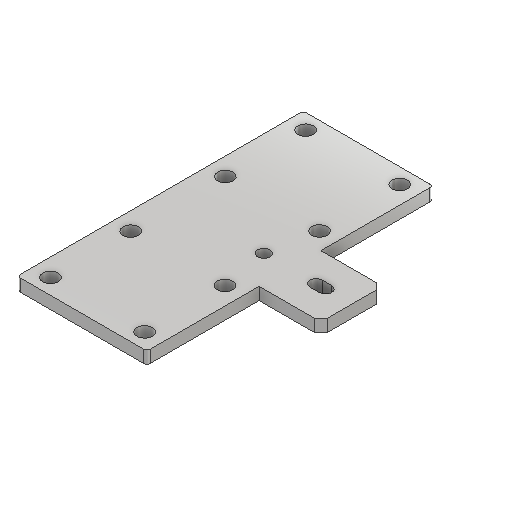
# Autodesk Inventor part: LC_ALU_4mm_X_End_Bearing_Side
Saved by Autodesk Inventor 2026.1 (Build 301233000, 233)
## iProperties
Created: 2017-05-25
Part Number: LC_ALU_4mm_X_End_Bearing_Side
Material: Ogólny
Document SubType Name: Modeling
Designer: Andrzej
Density: 1 g/cm^3
Appearance: Aluminium - ciemne
Mass: 16.3605 g
Surface Area: 100.28 cm^2
Volume: 16.3605 cm^3
Author: Andrzej
Autodesk Inventor part; units mm, degrees
ref_plane "YZ Plane" through (0, 0, 0) normal (1, 0, 0) x (0, 1, 0)
ref_plane "XZ Plane" through (0, 0, 0) normal (0, 1, 0) x (-1, 0, 0)
ref_plane "XY Plane" through (0, 0, 0) normal (0, 0, 1) x (1, 0, 0)
sketch "Szkic1" plane through (0, 0, 0) normal (0, 0, 1) x (1, 0, 0)
  line L0 (-10.2233, 17.3341) -> (-10.2233, -75.2659)
  line L1 (-10.2233, -75.2659) -> (31.7767, -75.2659)
  line L2 (-10.2233, 17.3341) -> (31.7767, 17.3341)
  line L3 (31.7767, 17.3341) -> (31.7767, -18.9659)
  line L4 (31.7767, -75.2659) -> (31.7767, -38.9659)
  line L5 (31.7767, -38.9659) -> (51.7767, -38.9659)
  line L6 (51.7767, -38.9659) -> (51.7767, -18.9659)
  line L7 (51.7767, -18.9659) -> (31.7767, -18.9659)
  line L8 (43.2767, -28.9659) -> (40.2767, -28.9659) construction
  line L9 (43.2767, -26.9659) -> (40.2767, -26.9659)
  line L10 (40.2767, -30.9659) -> (43.2767, -30.9659)
  arc A0 (43.2767, -30.9659) -> (43.2767, -26.9659) centre (43.2767, -28.9659) ccw
  arc A1 (40.2767, -26.9659) -> (40.2767, -30.9659) centre (40.2767, -28.9659) ccw
  point P0 (0, 0)
  point P1 (-4.4733, 12.3341)
  point P2 (26.0267, 12.3341)
  point P3 (-4.4733, -13.6659)
  point P4 (26.0267, -13.6659)
  point P5 (-4.4733, -44.2659)
  point P6 (26.0267, -44.2659)
  point P7 (-4.4733, -70.2659)
  point P8 (26.0267, -70.2659)
  point P9 (41.7767, -28.9659)
  point P10 (23.2767, -28.9659)
  dimension "d0" = 92.6
  dimension "d1" = 42
  dimension "d2" = 20
  dimension "d3" = 20
  dimension "d4" = 36.3
  dimension "d39" = 5
  dimension "d40" = 5
  dimension "d41" = 5
  dimension "d42" = 5
  dimension "d43" = 5.75
  dimension "d44" = 5.75
  dimension "d45" = 42
  dimension "d46" = 5.75
  dimension "d47" = 5.75
  dimension "d48" = 5.75
  dimension "d49" = 5.75
  dimension "d50" = 36.3
  dimension "d51" = 5.75
  dimension "d52" = 5.75
  dimension "d60" = 26
  dimension "d61" = 26
  dimension "d62" = 26
  dimension "d63" = 26
  dimension "d65" = 10
  dimension "d66" = 10
  dimension "d74" = 1.5
  dimension "d75" = 4
  dimension "d76" = 33.5
  dimension "d77" = 10
  constraints: 24 end point, 4 point on circle, 4 tangent, 3 horizontal, 3 perpendicular, 3 vertical, 2 centre point, 1 midpoint, 1 parallel
  measures "d0" distance of L0.start L0.end
  measures "d1" distance of L0.end L1.end
  measures "d2" distance between parallel lines of L5 L7
  measures "d3" distance of L6.end L3.end
  measures "d4" distance between parallel lines of L2 L7
  measures "d39" distance from line of L2 point (-4.473, 12.334)
  measures "d40" distance from line of L2 point (26.027, 12.334)
  measures "d41" distance from line of L1 point (-4.473, -70.266)
  measures "d42" distance from line of L1 point (26.027, -70.266)
  measures "d43" distance from line of L0 point (-4.473, 12.334)
  measures "d44" distance from line of L3 point (26.027, 12.334)
  measures "d45" distance between parallel lines of L0 L3
  measures "d46" distance from line of L3 point (26.027, -13.666)
  measures "d47" distance from line of L0 point (-4.473, -13.666)
  measures "d48" distance from line of L0 point (-4.473, -44.266)
  measures "d49" distance from line of L0 point (-4.473, -70.266)
  measures "d50" distance of L1.end L4.end
  measures "d51" distance from line of L4 point (26.027, -70.266)
  measures "d52" distance from line of L4 point (26.027, -44.266)
  measures "d60" distance of point (-4.473, 12.334) point (-4.473, -13.666)
  measures "d61" distance of point (26.027, 12.334) point (26.027, -13.666)
  measures "d62" distance of point (26.027, -70.266) point (26.027, -44.266)
  measures "d63" distance of point (-4.473, -70.266) point (-4.473, -44.266)
  measures "d65" distance from line of L6 point (41.777, -28.966)
  measures "d66" distance from line of L7 point (41.777, -28.966)
  measures "d74" distance of point (41.777, -28.966) L8.end
  measures "d75" diameter of A1
  measures "d76" distance from line of L0 point (23.277, -28.966)
  measures "d77" distance from line of L7 point (23.277, -28.966)
extrude "Wyciągnięcie proste1" add sketch "Szkic1" along normal blind 4
chamfer "Faza1" distance 2 angle 45 2 edges at (51.7767, -18.9659, 2) (51.7767, -38.9659, 2)
hole "Otwór3" at (-4.4733, 12.3341, 0) at (26.0267, 12.3341, 0) at (-4.4733, -13.6659, 0) at (26.0267, -13.6659, 0) at (-4.4733, -44.2659, 0) at (26.0267, -44.2659, 0) at (-4.4733, -70.2659, 0) at (26.0267, -70.2659, 0) direction (0, 0, 1) diameter 5 end through all
fillet "Zaokrąglenie1" radius 1 4 edges at (31.7767, 17.3341, 2) (-10.2233, 17.3341, 2) (31.7767, -75.2659, 2) (-10.2233, -75.2659, 2)
hole "Otwór5" at (41.7767, -28.9659, 0) at (23.2767, -28.9659, 0) direction (0, 0, 1) diameter 4 end through all
equation "\"d4\" = -0.5 * d2 + 0.5 * d0"
equation "\"d39\" = d41"
equation "\"d40\" = d41"
equation "\"d42\" = d41"
equation "\"d44\" = d43"
equation "\"d45\" = d1"
equation "\"d46\" = d43"
equation "\"d47\" = d43"
equation "\"d48\" = d43"
equation "\"d49\" = d43"
equation "\"d51\" = d43"
equation "\"d52\" = d43"
